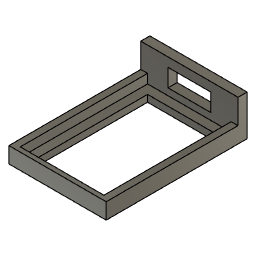
chargehold (Autodesk Fusion 360 design; units mm, degrees)
Autodesk Fusion 360 part; units mm, degrees
note: some values were not read from the file. Set by a fixed rule: which sketch regions a step uses.
sketch "Sketch1" plane through (0, 0, 0) normal (0, 1, 0) x (1, 0, 0)
  line L0 (0, 0) -> (17.5, 0)
  line L1 (17.5, 0) -> (17.5, -1.5)
  line L2 (17.5, -1.5) -> (0, -1.5)
  line L3 (0, -1.5) -> (0, 0)
  line L4 (4.25, -1.5) -> (13.25, -1.5)
  line L5 (13.25, -1.5) -> (13.25, -5)
  line L6 (13.25, -5) -> (4.25, -5)
  line L7 (4.25, -5) -> (4.25, -1.5)
  line L8 (4.05, -5.2) -> (13.45, -5.2)
  line L9 (13.45, -5.2) -> (13.45, -1.3)
  line L10 (13.45, -1.3) -> (4.05, -1.3)
  line L11 (4.05, -1.3) -> (4.05, -5.2)
  line L12 (-1.95, -7.2) -> (19.45, -7.2)
  line L13 (19.45, -7.2) -> (19.45, 1.7)
  line L14 (19.45, 1.7) -> (-1.95, 1.7)
  line L15 (-1.95, 1.7) -> (-1.95, -7.2)
  line L16 (19.45, 0.2) -> (-1.95, 0.2)
  line L17 (-1.95, 0.2) -> (-1.95, 1.7)
  line L18 (-1.95, 1.7) -> (19.45, 1.7)
  line L19 (19.45, 1.7) -> (19.45, 0.2)
  line L20 (-0.45, 0.2) -> (-1.95, 0.2)
  line L21 (-1.95, 0.2) -> (-1.95, -1.8)
  line L22 (-1.95, -1.8) -> (-0.45, -1.8)
  line L23 (-0.45, -1.8) -> (-0.45, 0.2)
  line L24 (19.45, -1.8) -> (17.95, -1.8)
  line L25 (17.95, -1.8) -> (17.95, 0.2)
  line L26 (17.95, 0.2) -> (19.45, 0.2)
  line L27 (19.45, 0.2) -> (19.45, -1.8)
  dimension "d1" = 17.5
  dimension "d2" = 1.5
  dimension "d3" = 9
  dimension "d4" = 3.5
  dimension "d5" = 4.25
  dimension "d10" = 0.2
  dimension "d11" = 0.2
  dimension "d12" = 0.2
  dimension "d13" = 0.2
  dimension "d14" = 6
  dimension "d15" = 6
  dimension "d16" = 2
  dimension "d17" = 3
  dimension "d18" = 21.4
  dimension "d19" = 1.5
  dimension "d20" = 0.2
  dimension "d21" = 1.5
  dimension "d22" = 2
  dimension "d23" = 1.5
  dimension "d24" = 2
  constraint horizontal L0
  constraint vertical L1
  constraint horizontal L2
  constraint vertical L3
  constraint coincident L0.start L3.end
  constraint horizontal L4
  constraint vertical L5
  constraint horizontal L6
  constraint vertical L7
  constraint coincident L2 L4.start
  constraint horizontal L8
  constraint vertical L9
  constraint horizontal L10
  constraint vertical L11
  constraint horizontal L12
  constraint vertical L13
  constraint horizontal L14
  constraint vertical L15
  constraint horizontal L16
  constraint vertical L17
  constraint horizontal L18
  constraint vertical L19
  constraint coincident L13 L16.start
  constraint horizontal L20
  constraint vertical L21
  constraint horizontal L22
  constraint vertical L23
  constraint coincident L16 L20.start
  constraint coincident L15 L21.end
  constraint horizontal L24
  constraint vertical L25
  constraint horizontal L26
  constraint vertical L27
  constraint coincident L13 L24.start
  constraint coincident L16 L25.end
  measures "d1" distance of L0.start L0.end
  measures "d2" distance of L0.start L2.end
  measures "d3" distance of L4.start L4.end
  measures "d4" distance of L4.start L6.end
  measures "d5" distance of L3 L7
  measures "d10" distance of L6 L8
  measures "d11" distance of L7 L11
  measures "d12" distance of L2 L10
  measures "d13" distance of L5 L9
  measures "d14" distance of L11 L15
  measures "d15" distance of L9 L13
  measures "d16" distance of L8 L12
  measures "d17" distance of L10 L14
  measures "d18" distance of L16.start L16.end
  measures "d19" distance of L16.start L13.end
  measures "d20" distance of L0 L16
  measures "d21" distance of L20.start L16.end
  measures "d22" distance of L20.start L22.end
  measures "d23" distance of L24.start L24.end
  measures "d24" distance of L24.start L16.start
extrude "Extrude1" add sketch "Sketch1" along normal blind 28 contours L0 L1 L2 L3 L9 L10 L11 | L2 L4 L9 L10 L11 makes body 1
extrude "Extrude2" add sketch "Sketch1" against normal blind 1.3 separate body contours L2 L4 L5 L6 L7 makes body 2
extrude "Extrude3" add sketch "Sketch1" along normal blind 2 separate body contours L0 L1 L2 L3 L9 L10 L11 | L12 L13 L15 L16 L22 L23 L24 L25 | L15 L16 L20 L21 L22 L23 | L13 L16 L24 L25 L26 L27 | L13 L14 L15 L16 L17 L18 L19 L20 L26 makes body 3
extrude "Extrude4" add sketch "Sketch1" against normal blind 28 contours L15 L16 L20 L21 L22 L23 | L13 L16 L24 L25 L26 L27 | L13 L14 L15 L16 L17 L18 L19 L20 L26 bodies 3
sketch "Sketch2" plane through (0, -28, 0) normal (0, -1, 0) x (1, 0, 0)
  line L0 (-1.95, 1.8) -> (-1.95, -1.7)
  line L1 (-1.95, -1.7) -> (19.45, -1.7)
  line L2 (19.45, -1.7) -> (19.45, 1.8)
  line L3 (19.45, 1.8) -> (17.95, 1.8)
  line L4 (17.95, 1.8) -> (17.95, -0.2)
  line L5 (17.95, -0.2) -> (-0.45, -0.2)
  line L6 (-0.45, -0.2) -> (-0.45, 1.8)
  line L7 (-0.45, 1.8) -> (-1.95, 1.8)
  line L8 (-1.95, 1.8) -> (19.45, 1.8)
  line L9 (19.45, 1.8) -> (19.45, -1.7)
  line L10 (19.45, -1.7) -> (-1.95, -1.7)
  line L11 (-1.95, -1.7) -> (-1.95, 1.8)
  constraint horizontal L8
  constraint vertical L9
  constraint horizontal L10
  constraint vertical L11
  constraint coincident L1.end L2.start
  constraint coincident L0.start L7.end
extrude "Extrude5" add sketch "Sketch2" along normal blind 1 bodies 3
sketch "Sketch3" plane through (0, 0, -0.2) normal (0, 0, 1) x (-1, 0, 0)
  line L0 (-17.95, 0) -> (0.45, 0)
  line L1 (0.45, 0) -> (0.45, 28)
  line L2 (0.45, 28) -> (-17.95, 28)
  line L3 (-17.95, 28) -> (-17.95, 0)
  line L4 (-1.55, 2) -> (-15.95, 2)
  line L5 (-15.95, 2) -> (-15.95, 26)
  line L6 (-15.95, 26) -> (-1.55, 26)
  line L7 (-1.55, 26) -> (-1.55, 2)
  dimension "d39" = 2
  dimension "d40" = 2
  dimension "d41" = 2
  dimension "d42" = 2
  constraint horizontal L4
  constraint vertical L5
  constraint horizontal L6
  constraint vertical L7
  measures "d39" distance of L3 L5
  measures "d40" distance of L0 L4
  measures "d41" distance of L1 L7
  measures "d42" distance of L2 L6
extrude "Extrude6" cut sketch "Sketch3" against normal blind 2 contours L4 L5 L6 L7 bodies 3
hidden bodies 1 2
